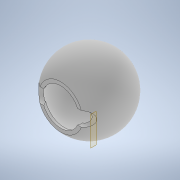
# Autodesk Inventor part: Part3
Saved by Autodesk Inventor 2022 (Build 260153000, 153)
## iProperties
Created: 2021-09-02
Part Number: Part3
Material: Generic
Document SubType Name: Modeling
Designer: tecware
Density: 1 g/cm^3
Appearance: Default
Author: tecware
## iProperties of the stored document marker_3DPrint.ipt
Created: 2021-09-02
Part Number: marker_3DPrint
Material: Generic
Document SubType Name: Modeling
Designer: tecware
Density: 1 g/cm^3
Appearance: Default
Author: tecware
Autodesk Inventor part; units mm, degrees
ref_plane "YZ Plane" through (0, 0, 0) normal (1, 0, 0) x (0, 1, 0)
ref_plane "XZ Plane" through (0, 0, 0) normal (0, 1, 0) x (-1, 0, 0)
ref_plane "XY Plane" through (0, 0, 0) normal (0, 0, 1) x (1, 0, 0)
sketch "Sketch1" plane through (0, 0, 0) normal (0, 1, 0) x (-1, 0, 0)
  spline S0 degree 2 poles (0, -5.7) (0.7354, -5.6783) (2.7683, -4.8041) (2.75, -2.4) knots -1 -1 -1 -0.79605 0 0 0 projected
  line L0 (-3.5, -2.4) -> (3.5, -2.4) projected
  line L1 (3.5, -2.4) -> (3.5, 0) projected
  line L2 (3.5, -1.5) -> (3.9, -1.5) projected
  arc A0 (3.9, -1.5) -> (4.3985, -1.1824) centre (3.9, -0.95) ccw projected
  line L3 (4.3985, -1.1824) -> (4.8592, -0.1943) projected
  arc A1 (5.0858, -0.05) -> (4.8592, -0.1943) centre (5.0858, -0.3) ccw projected
  line L4 (5.0858, -0.05) -> (5.2858, -0.05) projected
  line L5 (5.2858, -0.05) -> (5.5858, -0.05) projected
  line L6 (7.0858, -0.05) -> (5.5858, -0.05) projected
  circle A2 centre (0, -8) radius 10
  line L7 (0, -18) -> (0, 2)
  line L8 (3.5, -2.4) -> (0, -2.4)
  circle A3 centre (0, -2.4) radius 3.5
  arc A4 (3.5, -2.4) -> (5.0858, -0.05) centre (3.2203, -0.5012) ccw
  circle A5 centre (0, -2.4) radius 5.6025
  point P0 (6.0661, -0.05)
  point P1 (0, -8.0025)
  constraints: 4 end point, 4 point on circle, 2 centre point, 2 coincident, 1 horizontal alignment, 1 midpoint, 1 point on line, 1 vertical, 5 other
revolve "Revolution1" add sketch "Sketch1" angle 360 about axis through (0, 0, -18) along (0, 0, 1) contours A5 L4 L5 L6 A2 L7
shell "Shell1" thickness 1 removed faces 1 at (-2.801, -4.8515, -2.4695)
ref_plane "Work Plane1" through (10, 5.7735, 0.25) normal (1, 0, 0) x (0, -1, 0)
sketch "Sketch2" plane through (10, 5.7735, 0.25) normal (1, 0, 0) x (0, -1, 0)
  line L0 (10.8593, 0.3) -> (0.6877, 0.3) projected
  line L1 (3.3511, 0.3) -> (9, 0.3)
  line L2 (11.2109, 1.3) -> (0.3361, 1.3) projected
  line L3 (3.7735, 2.3) -> (7.7735, 2.3)
  line L4 (7.7735, 2.3) -> (7.7735, 0.3)
  line L5 (7.7735, 0.3) -> (3.7735, 0.3)
  line L6 (3.7735, 0.3) -> (3.7735, 2.3)
  line L7 (3.7735, 2.3) -> (7.7735, 0.3) construction
  line L8 (7.7735, 2.3) -> (3.7735, 0.3) construction
  point P0 (5.7735, 0.25)
  point P1 (5.7735, 1.3)
  dimension "d2" = 4
  constraints: 14 end point, 3 midpoint, 2 horizontal, 2 parallel, 2 point on line, 1 perpendicular
  measures "d2" distance of L4.end L5.end
extrude "Extrusion1" cut sketch "Sketch2" against normal through all
fillet "Fillet1" radius 2 4 edges at (7.117, 2, -2.05) (7.117, -2, -2.05) (-7.117, -2, -2.05) (-7.117, 2, -2.05)
body "Solid1"
